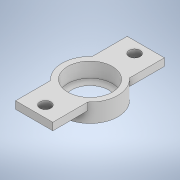
# Autodesk Inventor part: Ball houder plaat
Saved by Autodesk Inventor 2022 (Build 260153000, 153)
## iProperties
Created: 2022-11-19
Part Number: Ball houder plaat
Material: Generic
Document SubType Name: Modeling
Designer: Kilian De Ruyck
Density: 1 g/cm^3
Appearance: Default
Author: Kilian De Ruyck
Autodesk Inventor part; units mm, degrees
ref_plane "YZ Plane" through (0, 0, 0) normal (1, 0, 0) x (0, 1, 0)
ref_plane "XZ Plane" through (0, 0, 0) normal (0, 1, 0) x (-1, 0, 0)
ref_plane "XY Plane" through (0, 0, 0) normal (0, 0, 1) x (1, 0, 0)
sketch "Sketch1" plane through (0, 0, 0) normal (0, 1, 0) x (-1, 0, 0)
  circle A0 centre (0, 0) radius 5
  circle A1 centre (0, 0) radius 7.5
  dimension "d0" = 10
  dimension "d1" = 15
  constraints: 2 centre point, 2 coincident
  measures "d0" diameter of A0
  measures "d1" diameter of A1
extrude "Extrusion1" add sketch "Sketch1" along normal blind 14
sketch "Sketch2" plane through (0, 14, 0) normal (0, 1, 0) x (1, 0, 0)
  circle A0 centre (0, 0) radius 6
  dimension "d4" = 12
  constraints: 1 centre point, 1 coincident
  measures "d4" diameter of A0
extrude "Extrusion2" cut sketch "Sketch2" against normal blind 12
sketch "Sketch3" plane through (0, 14, 0) normal (0, 1, 0) x (1, 0, 0)
  circle A0 centre (0, 0) radius 7.5
  circle A1 centre (0, 0) radius 5.7555
  constraints: 2 centre point, 2 coincident
extrude "Extrusion3" cut sketch "Sketch3" against normal blind 2
sketch "Sketch4" plane through (0, 12, 0) normal (0, 1, 0) x (1, 0, 0)
  circle A0 centre (0, 0) radius 7.5
  line L0 (0, 0) -> (5, 0)
  line L1 (5, 0) -> (5, 15)
  line L2 (5, 15) -> (0, 15)
  line L3 (0, 15) -> (0, 0)
  line L4 (-5, 0) -> (-5, 15)
  line L5 (-5, 15) -> (0, 15)
  line L6 (5, 0) -> (5, -15)
  line L7 (5, -15) -> (0, -15)
  line L8 (-5, 0) -> (-5, -15)
  line L9 (-5, -15) -> (0, -15)
  point P0 (5, -5.5902)
  point P1 (-5, -5.5902)
  point P2 (-5, 5.5902)
  point P3 (5, 5.5902)
  dimension "d9" = 5
  dimension "d10" = 15
  constraints: 20 end point, 5 symmetric about line, 2 parallel, 1 centre point, 1 coincident, 1 horizontal, 1 perpendicular
  measures "d9" distance of L2.end L1.end
  measures "d10" distance of L1.end L0.end
extrude "Extrusion4" add sketch "Sketch4" against normal blind 8 contours A0 L3 L2 L1 | L6 L7 L9 L8 A0 | A0 L4 L5 L3
sketch "Sketch5" plane through (0, 4, 0) normal (0, -1, 0) x (1, 0, 0)
  line L0 (-5, -5.5902) -> (-5, -15) projected
  line L1 (-5, 15) -> (-5, 5.5902) projected
  point P0 (0, 0)
  point P1 (0, -12)
  point P2 (0, 12)
  dimension "d13" = 12
  dimension "d14" = 12
  dimension "d15" = 5
  dimension "d16" = 5
  measures "d13" distance of point (0, 0) point (0, -12)
  measures "d14" distance of point (0, 12) point (0, 0)
  measures "d15" distance from line of L0 point (0, -12)
  measures "d16" distance from line of L1 point (0, 12)
hole "Hole1" at (0, 4, -12) at (0, 4, 12) direction (0, 1, 0) diameter 3 depth 2
sketch "Sketch6" plane through (0, 0, 0) normal (0, -1, 0) x (1, 0, 0)
  circle A0 centre (0, 0) radius 7.5
  constraints: 1 centre point, 1 coincident
extrude "Extrusion5" cut sketch "Sketch6" against normal blind 1
fillet "Fillet1" radius 2 1 edges at (5, 2, 0)
sketch "Sketch7" plane through (0, 12, 0) normal (0, 1, 0) x (1, 0, 0)
  line L0 (9.97, 16.2589) -> (-13.6487, 16.2589)
  line L1 (-13.6487, 16.2589) -> (-13.6487, -18.2286)
  line L2 (-13.6487, -18.2286) -> (9.97, -18.2286)
  line L3 (9.97, -18.2286) -> (9.97, 16.2589)
  point P0 (0, 0)
  constraints: 8 end point, 2 parallel, 1 horizontal, 1 perpendicular
extrude "Extrusion6" cut sketch "Sketch7" against normal blind 6
equation "\"d14\" = d13"
equation "\"d16\" = d15"
body "Solid1"
